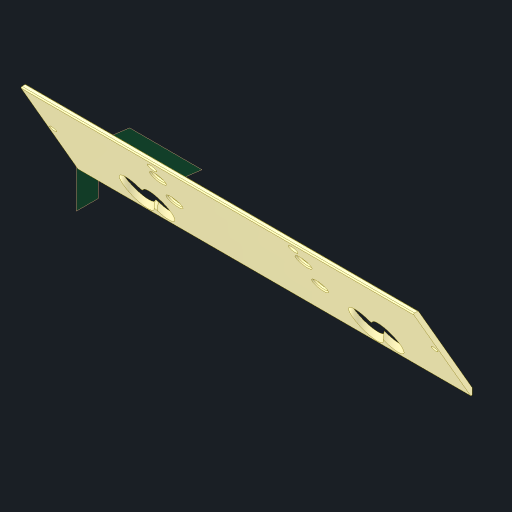
# Autodesk Inventor part: front
Saved by Autodesk Inventor 2023 (Build 270158000, 158)
## iProperties
Created: 2024-05-26
Part Number: front
Material: Nylon 6
Document SubType Name: Modeling
Designer: szymo
Density: 1.12 g/cm^3
Appearance: Nylon 6
Mass: 18.6267 g
Surface Area: 186.523 cm^2
Volume: 16.631 cm^3
TOTAL MASS: 0.0
Author: szymo
Autodesk Inventor part; units mm, degrees
ref_plane "YZ Plane" through (0, 0, 0) normal (1, 0, 0) x (0, 1, 0)
ref_plane "XZ Plane" through (0, 0, 0) normal (0, 1, 0) x (-1, 0, 0)
ref_plane "XY Plane" through (0, 0, 0) normal (0, 0, 1) x (1, 0, 0)
ref_plane "Work Plane1" through (-178, 0.5, -3.5) normal (-1, 0, 0) x (0, 0, 1)
sketch "Sketch1" plane through (-178, 0.5, -3.5) normal (-1, 0, 0) x (0, 0, 1)
  line L0 (3.5, 3.5) -> (-1, 3.5) projected
  line L1 (-1, 3.5) -> (-1, -0.5) projected
  line L2 (-1, -0.5) -> (-4.5, -0.5) projected
  line L3 (-4.5, -0.5) -> (-4.5, -14.5) projected
  line L4 (-4.5, -14.5) -> (4.5, -0.5) projected
  line L5 (4.5, -0.5) -> (3.5, -0.5) projected
  line L6 (3.5, -0.5) -> (3.5, 3.5) projected
  circle A0 centre (8.5, 158.5) radius 3 projected
  circle A1 centre (8.5, 158.5) radius 25
  circle A2 centre (13, 116) radius 15 projected
  line L7 (3.5, 3.5) -> (28, 45.9352)
  line L8 (3.5, -0.5) -> (30.3094, 45.9352)
  line L9 (30.3094, 45.9352) -> (28, 45.9352)
  line L10 (28, 45.9352) -> (28, 130) projected
  dimension "d0" = 50
  dimension "d1" = 30
  dimension "d3" = 2
  dimension "d4" = 4
  dimension "d5" = 2.3094
  constraints: 6 end point, 2 point on line, 1 centre point, 1 coincident, 1 horizontal, 1 parallel
  measures "d0" diameter of A1
  measures "d1" angle of L7 L6
  measures "d3" distance between parallel lines of L8 L7
  measures "d4" distance of L8.start L0.start
  measures "d5" distance of L7.end L8.end
ref_plane "Work Plane2" through (0, -14, -8) normal (1, 0, 0) x (0, 1, 0)
extrude "Extrusion1" add sketch "Sketch1" against normal up to surface (178 mm away) contours L7 L9 L8 L6
ref_plane "Work Plane3" through (-141.1151, 26.996, 4.2847) normal (0, -0.9925462, 0.1218693) x (1, 0, 0)
sketch "Sketch3" plane through (-141.1151, 26.996, 4.2847) normal (0, -0.9925462, 0.1218693) x (1, 0, 0)
  line L0 (89.3087, 5.4518) -> (89.3087, -5.4534)
  spline S0 degree 3 poles (89.3087, -5.4534) (89.308, -5.5772) (89.3587, -5.6989) (89.4451, -5.7853) (89.4649, -5.8051) (89.4865, -5.823) (89.5096, -5.8388) (89.529, -5.8521) (89.5494, -5.864) (89.5707, -5.8743) (89.5866, -5.882) (89.603, -5.8889) (89.6197, -5.8948) (89.6699, -5.9125) (89.7231, -5.9218) (89.7769, -5.9215) knots 0 0 0 0 0.5 0.5 0.5 0.614375 0.614375 0.614375 0.710781 0.710781 0.710781 0.783086 0.783086 0.783086 1 1 1 1
  line L1 (89.7769, -5.9215) -> (118.6836, -5.9215)
  spline S1 degree 3 poles (118.6836, -5.9215) (118.8077, -5.9222) (118.9296, -5.8713) (119.1025, -5.6977) (119.1524, -5.5758) (119.1517, -5.4518) knots 0 0 0 0 0.5 0.5 1 1 1 1
  line L2 (119.1517, -5.4518) -> (119.1517, 5.4534)
  spline S2 degree 3 poles (119.1517, 5.4534) (119.1524, 5.5775) (119.1015, 5.6994) (118.9279, 5.8723) (118.806, 5.9222) (118.682, 5.9215) knots 0 0 0 0 0.5 0.5 1 1 1 1
  line L3 (118.682, 5.9215) -> (89.7769, 5.9215)
  spline S3 degree 3 poles (89.7769, 5.9215) (89.6527, 5.9222) (89.5308, 5.8713) (89.3579, 5.6977) (89.308, 5.5758) (89.3087, 5.4518) knots 0 0 0 0 0.5 0.5 1 1 1 1
  circle A0 centre (90.8511, -4.3791) radius 0.5
  circle A1 centre (90.8511, 4.3791) radius 0.5
  circle A2 centre (117.6093, 4.3791) radius 0.5
  circle A3 centre (117.6093, -4.3791) radius 0.5
  arc A4 (104.4919, -1.4512) -> (104.4113, -1.5218) centre (104.5073, -1.55) ccw
  arc A5 (104.4113, 1.5218) -> (104.4113, -1.5218) centre (99.2302, 0) ccw
  arc A6 (104.4113, 1.5218) -> (104.4919, 1.4512) centre (104.5073, 1.55) ccw
  arc A7 (104.4919, 1.4512) -> (104.5716, 1.519) centre (104.4765, 1.55) ccw
  arc A8 (104.5716, -1.519) -> (104.5716, 1.519) centre (109.2302, 0) ccw
  arc A9 (104.5716, -1.519) -> (104.4919, -1.4512) centre (104.4765, -1.55) ccw
  line L4 (-14.6217, 5.4518) -> (-14.6217, -5.4534)
  spline S4 degree 3 poles (-14.6217, -5.4534) (-14.6224, -5.5772) (-14.5717, -5.6989) (-14.4853, -5.7853) (-14.4655, -5.8051) (-14.4439, -5.823) (-14.4208, -5.8388) (-14.4014, -5.8521) (-14.3809, -5.864) (-14.3597, -5.8743) (-14.3438, -5.882) (-14.3274, -5.8889) (-14.3107, -5.8948) (-14.2605, -5.9125) (-14.2073, -5.9218) (-14.1535, -5.9215) knots 0 0 0 0 0.5 0.5 0.5 0.614375 0.614375 0.614375 0.710781 0.710781 0.710781 0.783086 0.783086 0.783086 1 1 1 1
  line L5 (-14.1535, -5.9215) -> (14.7532, -5.9215)
  spline S5 degree 3 poles (14.7532, -5.9215) (14.8773, -5.9222) (14.9992, -5.8713) (15.1721, -5.6977) (15.222, -5.5758) (15.2213, -5.4518) knots 0 0 0 0 0.5 0.5 1 1 1 1
  line L6 (15.2213, -5.4518) -> (15.2213, 5.4534)
  spline S6 degree 3 poles (15.2213, 5.4534) (15.222, 5.5775) (15.1711, 5.6994) (14.9975, 5.8723) (14.8757, 5.9222) (14.7516, 5.9215) knots 0 0 0 0 0.5 0.5 1 1 1 1
  line L7 (14.7516, 5.9215) -> (-14.1535, 5.9215)
  spline S7 degree 3 poles (-14.1535, 5.9215) (-14.2776, 5.9222) (-14.3996, 5.8713) (-14.5725, 5.6977) (-14.6224, 5.5758) (-14.6217, 5.4518) knots 0 0 0 0 0.5 0.5 1 1 1 1
  circle A10 centre (-13.0792, -4.3791) radius 0.5
  circle A11 centre (-13.0792, 4.3791) radius 0.5
  circle A12 centre (13.6789, 4.3791) radius 0.5
  circle A13 centre (13.6789, -4.3791) radius 0.5
  arc A14 (0.5615, -1.4512) -> (0.4809, -1.5218) centre (0.5769, -1.55) ccw
  arc A15 (0.4809, 1.5218) -> (0.4809, -1.5218) centre (-4.7002, 0) ccw
  arc A16 (0.4809, 1.5218) -> (0.5615, 1.4512) centre (0.5769, 1.55) ccw
  arc A17 (0.5615, 1.4512) -> (0.6412, 1.519) centre (0.5461, 1.55) ccw
  arc A18 (0.6412, -1.519) -> (0.6412, 1.519) centre (5.2998, 0) ccw
  arc A19 (0.6412, -1.519) -> (0.5615, -1.4512) centre (0.5461, -1.55) ccw
  circle A20 centre (99.2302, 0) radius 5.4
  circle A21 centre (109.2302, 0) radius 4.9
  circle A22 centre (-4.7002, 0) radius 5.4
  circle A23 centre (5.2998, 0) radius 4.9
  arc A24 (0.5923, 3.0331) -> (0.5923, -3.0331) centre (-4.7002, 0) ccw
  arc A25 (0.5923, -3.0331) -> (0.5923, 3.0331) centre (5.2998, 0) ccw
  arc A26 (104.5227, -3.0331) -> (104.5227, 3.0331) centre (109.2302, 0) ccw
  arc A27 (104.5227, 3.0331) -> (104.5227, -3.0331) centre (99.2302, 0) ccw
  point P0 (141.1151, -7.5427)
  point P1 (104.4877, 1.2324)
  point P2 (104.4113, 1.5218)
  point P3 (104.4113, -1.5218)
  point P4 (104.4877, -1.2324)
  point P5 (104.5716, -1.519)
  point P6 (104.5716, 1.519)
  point P7 (0.5573, 1.2324)
  point P8 (0.4809, 1.5218)
  point P9 (0.4809, -1.5218)
  point P10 (0.5573, -1.2324)
  point P11 (0.6412, -1.519)
  point P12 (0.6412, 1.519)
  dimension "d19" = 0.7
  dimension "d20" = 0.7
  constraints: 8 centre point, 8 point on circle, 4 coincident, 4 concentric, 2 other
  measures "d19" radial gap between concentric circles of A18 A25
  measures "d20" radial gap between concentric circles of A5 A27
extrude "Extrusion2" cut sketch "Sketch3" along normal up to next contours A27 L3 | L3 A27 A26 L1 | L1 A27 | A4 A20 A21 A9 | A5 A20 A21 | A21 A20 A8 | A6 A7 A21 A20 | A21 A20 | A24 L7 | L7 A24 A25 L5 | L5 A24 | A14 A22 A23 A19 | A15 A22 A23 | A23 A22 A18 | A16 A17 A23 A22 | A23 A22
fillet "Fillet1" radius 1 3 edges at (-140.5228, 16.868, 8.5841) (-140.5228, 8.1387, 3.5442) (-36.5924, 16.868, 8.5841)
sketch "Sketch4" plane through (-178, 46.4352, 26.8094) normal (0, -0.5, 0.8660254) x (1, 0, 0)
  line L0 (5, -23) -> (5, -26) projected
  line L1 (3, -2.3094) -> (3, -21) projected
  line L2 (0, -1.1547) -> (4, -1.1547) projected
  line L3 (0, -47.8453) -> (0, -1.1547) projected
  line L4 (0, -47.8453) -> (3, -47.8453) projected
  line L5 (3, -46.6906) -> (3, -47.8453) projected
  line L6 (175, -28) -> (175, -43.1547) projected
  line L7 (178, -47.8453) -> (175, -47.8453) projected
  line L8 (178, -47.8453) -> (178, -1.1547) projected
  line L9 (178, -1.1547) -> (174, -1.1547) projected
  line L10 (175, -2.3094) -> (175, -21) projected
  line L11 (173, -23) -> (173, -26) projected
  arc A0 (5, -23) -> (4, -22) centre (4, -23) ccw projected
  arc A1 (3, -21) -> (4, -22) centre (4, -21) ccw projected
  ellipse E0 centre (4, -2.3094) end of major axis (4, -1.1547) minor radius 1 (4, -1.1547) -> (3, -2.3094) ccw projected
  ellipse E1 centre (8, -46.6906) end of major axis (8, -40.9171) minor radius 5 (3.1753, -45.1754) -> (3, -46.6906) ccw projected
  ellipse E2 centre (6, -43.1547) end of major axis (6, -49.1547) minor radius 3 (3, -43.1547) -> (3.1753, -45.1754) ccw projected
  arc A2 (4, -27) -> (3, -28) centre (4, -28) ccw projected
  arc A3 (4, -27) -> (5, -26) centre (4, -26) ccw projected
  circle A4 centre (2.5, -24.5) radius 1.75 projected
  line L12 (3, -28) -> (3, -43.1547) projected
  arc A5 (174, -22) -> (173, -23) centre (174, -23) ccw projected
  arc A6 (173, -26) -> (174, -27) centre (174, -26) ccw projected
  arc A7 (175, -28) -> (174, -27) centre (174, -28) ccw projected
  ellipse E3 centre (174, -2.3094) end of major axis (174, -1.1547) minor radius 1 (175, -2.3094) -> (174, -1.1547) ccw projected
  arc A8 (174, -22) -> (175, -21) centre (174, -21) ccw projected
  circle A9 centre (175.5, -24.5) radius 1.75 projected
  ellipse E4 centre (172, -43.1547) end of major axis (172, -49.1547) minor radius 3 (174.8247, -45.1754) -> (175, -43.1547) ccw projected
  ellipse E5 centre (170, -46.6906) end of major axis (170, -40.9171) minor radius 5 (175, -46.6906) -> (174.8247, -45.1754) ccw projected
  line L13 (175, -46.6906) -> (175, -47.8453) projected
  arc A10 (118.5, -1.9585) -> (117.5, -3.6906) centre (119.5, -3.6906) ccw projected
  line L14 (117.5, -3.6906) -> (117.5, -6.7624) projected
  arc A11 (117.5, -6.7624) -> (118.5, -8.4944) centre (119.5, -6.7624) ccw projected
  arc A12 (119.5, -10.2265) -> (118.5, -8.4944) centre (117.5, -10.2265) ccw projected
  line L15 (119.5, -10.2265) -> (119.5, -33.2065) projected
  line L16 (119.5, -33.2065) -> (124.5, -33.2065) projected
  line L17 (124.5, -1.1547) -> (124.5, -33.2065) projected
  line L18 (124.5, -1.1547) -> (119.2716, -1.1547) projected
  arc A13 (118.5, -1.9585) -> (119.2716, -1.1547) centre (117.5, -0.2265) ccw projected
  circle A14 centre (121, -5.2265) radius 2.3 projected
  circle A15 centre (122, -27.626) radius 1.75 projected
  circle A16 centre (122, -12.626) radius 1.75 projected
  arc A17 (60.5, -3.6906) -> (59.5, -1.9585) centre (58.5, -3.6906) ccw projected
  arc A18 (58.7284, -1.1547) -> (59.5, -1.9585) centre (60.5, -0.2265) ccw projected
  line L19 (53.5, -1.1547) -> (58.7284, -1.1547) projected
  line L20 (53.5, -1.1547) -> (53.5, -33.2065) projected
  line L21 (58.5, -33.2065) -> (53.5, -33.2065) projected
  line L22 (58.5, -10.2265) -> (58.5, -33.2065) projected
  arc A19 (59.5, -8.4944) -> (58.5, -10.2265) centre (60.5, -10.2265) ccw projected
  arc A20 (59.5, -8.4944) -> (60.5, -6.7624) centre (58.5, -6.7624) ccw projected
  line L23 (60.5, -3.6906) -> (60.5, -6.7624) projected
  circle A21 centre (57, -5.2265) radius 2.3 projected
  circle A22 centre (56, -27.626) radius 1.75 projected
  circle A23 centre (56, -12.626) radius 1.75 projected
  point P0 (178, -53.6188)
  point P1 (3, -40.6533)
  constraints: 6 coincident, 6 other
hole "srobkiSrodek" at (-122, 22.5104, 12.9964) at (-122, 35.5008, 20.4964) at (-56, 22.5104, 12.9964) at (-56, 35.5008, 20.4964) direction (0, 0.5, -0.8660254) diameter 3.1 end through all counterbore diameter 6 counterbore depth 1.2 clearance for "Countersunk Raised Head Screw ISO 2010/7047" size "M2.5" standard "ISO"
sketch "Sketch6" plane through (-178, 46.4352, 26.8094) normal (0, -0.5, 0.8660254) x (1, 0, 0)
  circle A0 centre (57, -5.2265) radius 2.3 projected
  circle A1 centre (121, -5.2265) radius 2.3 projected
  point P0 (178, -53.6188)
  constraints: 2 coincident
hole "czulki" at (-57, 41.909, 24.1962) at (-121, 41.909, 24.1962) direction (0, 0.5, -0.8660254) diameter 4 end through all
sketch "Sketch7" plane through (-178, 46.4352, 26.8094) normal (0, -0.5, 0.8660254) x (1, 0, 0)
  circle A0 centre (2.5, -24.5) radius 1.75 projected
  arc A1 (4, -27) -> (5, -26) centre (4, -26) ccw projected
  line L0 (5, -23) -> (5, -26) projected
  arc A2 (5, -23) -> (4, -22) centre (4, -23) ccw projected
  arc A3 (3, -21) -> (4, -22) centre (4, -21) ccw projected
  line L1 (3, -2.3094) -> (3, -21) projected
  ellipse E0 centre (4, -2.3094) end of major axis (4, -1.1547) minor radius 1 (4, -1.1547) -> (3, -2.3094) ccw projected
  line L2 (0, -1.1547) -> (4, -1.1547) projected
  line L3 (0, -47.8453) -> (0, -1.1547) projected
  line L4 (0, -47.8453) -> (3, -47.8453) projected
  line L5 (3, -46.6906) -> (3, -47.8453) projected
  ellipse E1 centre (8, -46.6906) end of major axis (8, -40.9171) minor radius 5 (3.1753, -45.1754) -> (3, -46.6906) ccw projected
  ellipse E2 centre (6, -43.1547) end of major axis (6, -49.1547) minor radius 3 (3, -43.1547) -> (3.1753, -45.1754) ccw projected
  line L6 (3, -28) -> (3, -43.1547) projected
  arc A4 (4, -27) -> (3, -28) centre (4, -28) ccw projected
  circle A5 centre (175.5, -24.5) radius 1.75 projected
  arc A6 (173, -26) -> (174, -27) centre (174, -26) ccw projected
  arc A7 (175, -28) -> (174, -27) centre (174, -28) ccw projected
  line L7 (175, -28) -> (175, -43.1547) projected
  ellipse E3 centre (172, -43.1547) end of major axis (172, -49.1547) minor radius 3 (174.8247, -45.1754) -> (175, -43.1547) ccw projected
  ellipse E4 centre (170, -46.6906) end of major axis (170, -40.9171) minor radius 5 (175, -46.6906) -> (174.8247, -45.1754) ccw projected
  line L8 (175, -46.6906) -> (175, -47.8453) projected
  line L9 (178, -47.8453) -> (175, -47.8453) projected
  line L10 (178, -47.8453) -> (178, -1.1547) projected
  line L11 (178, -1.1547) -> (174, -1.1547) projected
  ellipse E5 centre (174, -2.3094) end of major axis (174, -1.1547) minor radius 1 (175, -2.3094) -> (174, -1.1547) ccw projected
  line L12 (175, -2.3094) -> (175, -21) projected
  arc A8 (174, -22) -> (175, -21) centre (174, -21) ccw projected
  arc A9 (174, -22) -> (173, -23) centre (174, -23) ccw projected
  line L13 (173, -23) -> (173, -26) projected
  point P0 (178, -53.6188)
  constraints: 2 coincident, 6 other
hole "srubkiBoki" at (-2.5, 25.2176, 14.5594) at (-175.5, 25.2176, 14.5594) direction (0, 0.5, -0.8660254) diameter 2.9 end through all clearance for "Countersunk Flat Head Screw ISO 2009/7046" size "M2.5" standard "ISO"
chamfer "Chamfer1" distance 0.5 angle 45 4 edges at (-122, 38.0989, 21.9964) (-122, 25.1085, 14.4964) (-56, 25.1085, 14.4964) (-56, 38.0989, 21.9964)
fillet "Fillet2" radius 0.4 4 edges at (-89, 0, 0) (-89, 4, 0) (-89, 46.4352, 24.5) (-89, 46.4352, 26.8094)
body "Solid1"
